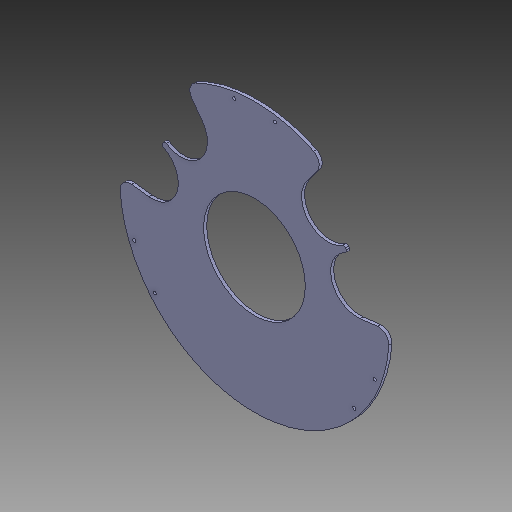
# Autodesk Inventor part: Диск_фиксирующий
Saved by Autodesk Inventor 2022 (Build 260153000, 153)
## iProperties
Created: 2025-01-10
Part Number: Диск_фиксирующий
Material: Типовые
Document SubType Name: Modeling
Designer: Ivan
Density: 1 g/cm^3
Appearance: Грифельно-синий
Mass: 108.493 g
Surface Area: 763.48 cm^2
Volume: 108.493 cm^3
Author: Ivan
Title: Диск_фиксирующий
Autodesk Inventor part; units mm, degrees
ref_plane "YZ Plane" through (0, 0, 0) normal (1, 0, 0) x (0, 1, 0)
ref_plane "XZ Plane" through (0, 0, 0) normal (0, 1, 0) x (-1, 0, 0)
ref_plane "XY Plane" through (0, 0, 0) normal (0, 0, 1) x (1, 0, 0)
sketch "Эскиз1" plane through (0, 0, 0) normal (0, 0, 1) x (1, 0, 0)
  circle A0 centre (0, 0) radius 104 construction
  line L0 (0, 0) -> (0, 166.3327) construction
  line L1 (0, 0) -> (122.2993, 70.6095) construction
  line L2 (0, 0) -> (95.803, 99.2069) construction
  line L3 (0, 0) -> (133.5999, 33.3102) construction
  circle A1 centre (72.2445, 74.8113) radius 26
  circle A2 centre (100.9108, 25.1599) radius 26
  circle A3 centre (0, 0) radius 132.5
  line L4 (51.4307, 90.3929) -> (68.6163, 113.3493)
  line L5 (88.543, 54.554) -> (110.8856, 72.5303)
  line L6 (91.5167, 49.4035) -> (118.2559, 59.7646)
  line L7 (103.9979, -0.6562) -> (132.4715, 2.7488)
  circle A4 centre (-72.2445, 74.8113) radius 26
  circle A5 centre (-100.9108, 25.1599) radius 26
  line L8 (-51.4307, 90.3929) -> (-68.6163, 113.3493)
  line L9 (-88.543, 54.554) -> (-110.8856, 72.5303)
  line L10 (-91.5167, 49.4035) -> (-118.2559, 59.7646)
  line L11 (-103.9979, -0.6562) -> (-132.4715, 2.7488)
  arc A6 (91.5167, 49.4035) -> (88.543, 54.554) centre (0, 0) ccw
  arc A7 (-88.543, 54.554) -> (-91.5167, 49.4035) centre (0, 0) ccw
  point P0 (-68.6163, 113.3493)
  point P1 (-110.8856, 72.5303)
  point P2 (-118.2559, 59.7646)
  point P3 (-132.4715, 2.7488)
  dimension "d0" = 208
  dimension "d1" = 52
  dimension "d2" = 32
  dimension "d3" = 60
  dimension "d4" = 265
  constraints: 24 end point, 22 point on circle, 10 symmetric about line, 8 centre point, 4 tangent, 3 equal radius, 2 coincident, 2 point on line, 1 vertical, 3 other
  measures "d0" diameter of A0
  measures "d1" diameter of A1
  measures "d2" angle of L3 L2
  measures "d3" angle of L0 L1
  measures "d4" diameter of A3
extrude "Выдавливание1" add sketch "Эскиз1" along normal mid plane 3 contours A1 A6 A2 L7 A3 L11 A5 A7 A4 L8 L4
fillet "Сопряжение1" radius 10 4 edges at (-68.6163, 113.3493, 0) (-132.4715, 2.7488, 0) (68.6163, 113.3493, 0) (132.4715, 2.7488, 0)
fillet "Сопряжение1" radius 2 4 edges at (88.543, 54.554, 0) (91.5167, 49.4035, 0) (-88.543, 54.554, 0) (-91.5167, 49.4035, 0)
sketch "Эскиз2" plane through (0, 0, 1.5) normal (0, 0, 1) x (1, 0, 0)
  circle A0 centre (20, 124.909) radius 1.95 construction
  circle A1 centre (20, 124.909) radius 1.6
  circle A2 centre (-20, 124.909) radius 1.6
  circle A3 centre (-20, 124.909) radius 1.6 projected
  point P0 (0, 0)
  dimension "d9" = 3.2
  constraints: 3 centre point, 2 coincident, 1 equal radius
  measures "d9" diameter of A2
extrude "Выдавливание2" cut sketch "Эскиз2" against normal through all
pattern_circular "Круговой массив1" count 3 over 360 about axis through (0, 0, -10) along (0, 0, 1) of "Выдавливание2"
sketch "Эскиз3" plane through (0, 0, 1.5) normal (0, 0, 1) x (1, 0, 0)
  circle A0 centre (0, 0) radius 50
  dimension "d15" = 100
  constraints: 1 centre point, 1 coincident
  measures "d15" diameter of A0
extrude "Выдавливание3" cut sketch "Эскиз3" against normal through all
